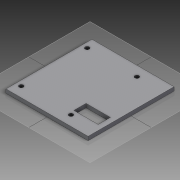
# Autodesk Inventor part: loader_frame
Saved by Autodesk Inventor 2013 (Build 170138000, 138)
## iProperties
Created: 2013-09-15
Part Number: loader_frame
Material: Generic
Document SubType Name: Modeling
Designer: Ian
Density: 1 g/cm^3
Mass: 117.522 g
Surface Area: 418.732 cm^2
Volume: 117.522 cm^3
Author: Ian
Autodesk Inventor part; units mm, degrees
ref_plane "YZ Plane" through (0, 0, 0) normal (1, 0, 0) x (0, 1, 0)
ref_plane "XZ Plane" through (0, 0, 0) normal (0, 1, 0) x (-1, 0, 0)
ref_plane "XY Plane" through (0, 0, 0) normal (0, 0, 1) x (1, 0, 0)
sketch "Sketch1" plane through (0, 0, 0) normal (0, 1, 0) x (-1, 0, 0)
  line L0 (-68.199, -71.3867) -> (68.199, -71.3867)
  line L1 (68.199, -71.3867) -> (68.199, 71.3867)
  line L2 (68.199, 71.3867) -> (-68.199, 71.3867)
  line L3 (-68.199, 71.3867) -> (-68.199, -71.3867)
  line L4 (-68.199, -71.3867) -> (68.199, 71.3867) construction
  line L5 (68.199, -71.3867) -> (-68.199, 71.3867) construction
  point P0 (0, 0)
  dimension "d0" = 136.398
  dimension "d1" = 142.7734
  constraints: 12 end point, 2 midpoint, 2 parallel, 1 horizontal, 1 perpendicular
  measures "d0" distance of L2.end L1.end
  measures "d1" distance of L1.end L0.end
extrude "Extrusion1" add sketch "Sketch1" along normal blind 6.35
sketch "Sketch2" plane through (0, 6.35, 0) normal (0, 1, 0) x (1, 0, 0)
  line L0 (-68.199, 71.3867) -> (-68.199, -71.3867) projected
  line L1 (-68.199, -71.3867) -> (68.199, -71.3867) projected
  line L2 (68.199, -71.3867) -> (68.199, 71.3867) projected
  line L3 (-59.436, -54.7751) -> (-59.436, 54.7497) construction
  line L4 (-59.436, 54.7497) -> (23.114, 54.7497) construction
  line L5 (23.114, 54.7497) -> (23.114, -54.7751) construction
  line L6 (23.114, -54.7751) -> (-59.436, -54.7751) construction
  line L7 (68.199, 71.3867) -> (-68.199, 71.3867) projected
  point P0 (0, 0)
  dimension "d4" = 8.763
  dimension "d5" = 16.6116
  dimension "d8" = 82.55
  dimension "d9" = 109.5248
  dimension "d17" = 16.637
  constraints: 8 end point, 4 coincident, 2 parallel, 2 perpendicular
  measures "d4" distance between parallel lines of L0 L3
  measures "d5" distance between parallel lines of L1 L6
  measures "d8" distance of L5.end L3.start
  measures "d9" distance of L4.end L5.end
  measures "d17" distance between parallel lines of L7 L4
hole "Hole1" at (-59.436, 6.35, -54.7497) at (23.114, 6.35, -54.7497) at (23.114, 6.35, 54.7751) at (-59.436, 6.35, 54.7751) direction (0, -1, 0) diameter 6.7818 end through all thread size "5/16-24 UNF" class "2B" standard "ANSI Unified Screw Threads"
sketch "Sketch3" plane through (0, 6.35, 0) normal (0, 1, 0) x (1, 0, 0)
  line L0 (59.563, -45.9867) -> (19.1008, -45.9867) projected
  line L1 (59.563, -25.6667) -> (59.563, -45.9867) projected
  line L2 (19.1008, -25.6667) -> (59.563, -25.6667) projected
  line L3 (19.1008, -45.9867) -> (19.1008, -25.6667) projected
  point P0 (0, 0)
extrude "Extrusion2" cut sketch "Sketch3" against normal up to next
body "Solid1"
